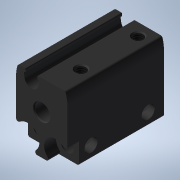
# Autodesk Inventor part: 5267300 AEN-S-6-5-I-A---(highH)
Saved by Autodesk Inventor 2025.1 (Build 291241000, 241)
## iProperties
Category: PARTsolutions
Company: FESTO
Created: 2025-06-16
Part Number: 5267300 AEN-S-6-5-I-A---(highH)
Material: Generic
Catalog Web Link: www.cadenas.de
Description: AEN-S---(H)-Compact cylinder
Vendor: FESTO
Document SubType Name: Modeling
Designer: psAdmin
Manufacturer: FESTO
Mass: 4.06306 g
Surface Area: 29.8936 cm^2
Volume: 4.06306 cm^3
Density: 1 g/cm^3
Appearance: PSOLRGB-175-175-175
PSOL_IDENT_0: {$CADENAS_DATA/23d-libs/festo/parts/a/aen/parts/aen_s_housing.prj},215 {VTYP=3D},{NB=5267300 AEN-S-6
PSOL_IDENT_1: -5-I-A---(highH)},{LINA=5267300 AEN-S-6-5-I-A---(highH)},{NN=AEN-S---(H)},{DATE=04.06.2025 19:32:15}
PSOL_IDENT_2: ,{GEOMDATE=23.08.2023 14:28:27},{VERSION=},{LINEID=30},{WBVAR=LODLEVEL},{WBNUMERIC=}  {NB=5267300 AE
PSOL_IDENT_3: N-S-6-5-I-A---(highH)},{LINA=5267300 AEN-S-6-5-I-A---(highH)},{KT=DUMMY},{TNR=5267300},{TYP=AEN-S-6-
PSOL_IDENT_4: 5-I-A},{LODDEST=mechanical},{LODLEVEL=high},{LODLEVELX='high', 'High', 'medium', 'Medium','low','Low'
PSOL_IDENT_5: },{BAU=S},{KDM=6},{HUB=5},{A=5.000},{SF=3.500},{E1=13.000},{E2=17.500},{ZB=27.500},{ZA=24.500},{L2=8
PSOL_IDENT_6: .100},{L3=10.000},{L4=7.000},{WL=2.700},{T=3.000},{KF=M2.5},{KFD=2.5},{P1=6.000},{P2=4.000},{P3=3.00
PSOL_IDENT_7: 0},{PL1=7.000},{PL2=3.000},{TG=7.000},{D1=5.800},{D2=3.300},{EE=M3},{EED=3.0},{MM=4.000},{WH=3.000}
NB: 5267300 AEN-S-6-5-I-A---(highH)
NN: AEN-S---(H)
NT: Compact cylinder
NBSYN: $TNR. $TYP.---($LODLEVEL.H)
LINA: 5267300 AEN-S-6-5-I-A---(highH)
CATALOG: Festo
TNR: 5267300
TYP: AEN-S-6-5-I-A
LODLEVEL: High
BAU: S
KDM: 6
HUB: 5
A: 5
SF: 3.5
E1: 13
E2: 17.5
ZB: 27.5
ZA: 24.5
L2: 8.1
L3: 10
L4: 7
WL: 2.7
T: 3
KF: M2.5
KFD: 2.5
P1: 6
P2: 4
P3: 3
PL1: 7
PL2: 3
TG: 7
D1: 5.8
D2: 3.3
EE: M3
EED: 3
MM: 4
WH: 3
SUPPLIER: FESTO
ARTICLENO: 5267300 AEN-S-6-5-I-A---(highH)
BOMINFO: 5267300 AEN-S-6-5-I-A---(highH)
CREATOR: CADENAS GmbH
Title: 5267300 AEN-S-6-5-I-A---(highH)
Author: Cadenas PARTsolutions
Comments: Compact cylinder
Autodesk Inventor part; units mm, degrees
sketch "Sketch_1" plane through (0, 0, 0) normal (0, 0, 1) x (1, 0, 0)
  arc A0 (-6.5, -9.5) -> (-6, -10) centre (-6, -9.5) ccw
  line L0 (-6, -10) -> (6, -10)
  arc A1 (6, -10) -> (6.5, -9.5) centre (6, -9.5) ccw
  line L1 (6.5, -9.5) -> (6.5, 4.8)
  arc A2 (6.5, 4.8) -> (6.1481, 7.1467) centre (-1.5, 4.8) ccw
  arc A3 (6.1481, 7.1467) -> (5.6701, 7.5) centre (5.6701, 7) ccw
  line L2 (5.6701, 7.5) -> (-0.9, 7.5)
  arc A4 (-0.9, 7.5) -> (-1.1, 7.3) centre (-0.9, 7.3) ccw
  line L3 (-1.1, 7.3) -> (-1.1, 6.9)
  arc A5 (-1.1, 6.9) -> (-0.8993, 6.7) centre (-0.9, 6.9) ccw
  arc A6 (-0.7, 6.4755) -> (-0.8993, 6.7) centre (-0.8985, 6.5) ccw
  line L4 (-0.7, 6.4755) -> (-0.824, 5.4709)
  arc A7 (-4.376, 5.4709) -> (-0.824, 5.4709) centre (-2.6, 5.69) ccw
  line L5 (-4.376, 5.4709) -> (-4.5, 6.4755)
  arc A8 (-4.3007, 6.7) -> (-4.5, 6.4755) centre (-4.3015, 6.5) ccw
  arc A9 (-4.3007, 6.7) -> (-4.1, 6.9) centre (-4.3, 6.9) ccw
  line L6 (-4.1, 6.9) -> (-4.1, 7.3)
  arc A10 (-4.1, 7.3) -> (-4.3, 7.5) centre (-4.3, 7.3) ccw
  line L7 (-4.3, 7.5) -> (-5.6701, 7.5)
  arc A11 (-5.6701, 7.5) -> (-6.1481, 7.1467) centre (-5.6701, 7) ccw
  arc A12 (-6.1481, 7.1467) -> (-6.5, 4.8) centre (1.5, 4.8) ccw
  line L8 (-6.5, 4.8) -> (-6.5, -9.5)
  constraints: 26 point on circle, 18 end point, 13 centre point
extrude "Extrusion1" add sketch "Sketch_1" against normal blind 24.5
sketch "Sketch_2" plane through (0, 0, 0) normal (0, 0, 1) x (1, 0, 0)
  line L0 (-8.5, -12) -> (8.5, -12)
  line L1 (8.5, -12) -> (8.5, -4.5174)
  line L2 (8.5, -4.5174) -> (6.5, -4.5174)
  arc A0 (5.75, -4.9504) -> (6.5, -4.5174) centre (6, -4.5174) ccw
  line L3 (5.75, -4.9504) -> (4.95, -4.4885)
  arc A1 (4.95, -4.4885) -> (1.2785, -8.8641) centre (3.5, -7) ccw
  line L4 (1.2785, -8.8641) -> (1.5424, -9.1786)
  arc A2 (1.1594, -10) -> (1.5424, -9.1786) centre (1.1594, -9.5) ccw
  line L5 (1.1594, -10) -> (-1.1594, -10)
  arc A3 (-1.5424, -9.1786) -> (-1.1594, -10) centre (-1.1594, -9.5) ccw
  line L6 (-1.5424, -9.1786) -> (-1.2785, -8.8641)
  arc A4 (-1.2785, -8.8641) -> (-4.95, -4.4885) centre (-3.5, -7) ccw
  line L7 (-4.95, -4.4885) -> (-5.75, -4.9504)
  arc A5 (-6.5, -4.5174) -> (-5.75, -4.9504) centre (-6, -4.5174) ccw
  line L8 (-6.5, -4.5174) -> (-8.5, -4.5174)
  line L9 (-8.5, -4.5174) -> (-8.5, -12)
  constraints: 20 end point, 12 point on circle, 6 centre point
extrude "Extrusion2" cut sketch "Sketch_2" against normal blind 3
sketch "Sketch3" plane through (0, 0, -24.5) normal (0, 0, -1) x (-1, 0, 0)
  point P0 (-3.5, -7)
hole "Hole1" at (3.5, -7, -24.5) direction (0, 0, 1) diameter 3.3 depth 24.5
sketch "Sketch4" plane through (0, 0, -24.5) normal (0, 0, -1) x (-1, 0, 0)
  point P0 (3.5, -7)
hole "Hole2" at (-3.5, -7, -24.5) direction (0, 0, 1) diameter 3.3 depth 24.5
sketch "Sketch5" plane through (6.5, -9.5, -24.5) normal (1, 0, 0) x (0, 0, -1)
  point P0 (-18.5, 2.5)
hole "Hole3" at (6.5, -7, -6) direction (-1, 0, 0) diameter 3.3 depth 13
sketch "Sketch6" plane through (6.5, -9.5, -24.5) normal (1, 0, 0) x (0, 0, -1)
  point P0 (-4, 2.5)
hole "Hole4" at (6.5, -7, -20.5) direction (-1, 0, 0) diameter 3.3 depth 13
sketch "Sketch7" plane through (-0.9, 7.5, 0) normal (0, 1, 0) x (1, 0, 0)
  point P0 (3.9, 7)
hole "Hole5" at (3, 7.5, -7) direction (0, -1, 0) diameter 2.459 depth 3.8 countersink diameter 3 countersink angle 90 thread size "M3x0.5" class "6H" standard "ISO Metric profile"
sketch "Sketch8" plane through (-0.9, 7.5, 0) normal (0, 1, 0) x (1, 0, 0)
  point P0 (3.9, 21.5)
hole "Hole6" at (3, 7.5, -21.5) direction (0, -1, 0) diameter 2.459 depth 3.8 countersink diameter 3 countersink angle 90 thread size "M3x0.5" class "6H" standard "ISO Metric profile"
sketch "Sketch_9" plane through (0, 0, 0) normal (1, 0, 0) x (0, 1, 0)
  line L0 (0, -24.5) -> (0, -24.1)
  line L1 (0, -24.1) -> (3.3845, -24.1)
  line L2 (3.3845, -24.1) -> (3.5, -23.9)
  line L3 (3.5, -23.9) -> (3.5, -24.4)
  line L4 (3.5, -24.4) -> (3.6, -24.5)
  line L5 (3.6, -24.5) -> (0, -24.5)
  line L6 (0, -24.5) -> (0, -24.1)
  constraints: 14 end point
revolve "Revolution1" cut sketch "Sketch_9" angle 360 about axis through (0, 0, -24.5) along (0, 0, -1)
sketch "Sketch_10" plane through (0, 0, 0) normal (1, 0, 0) x (0, 1, 0)
  line L0 (0, -22.1) -> (0, 0)
  line L1 (0, 0) -> (2.1732, 0)
  line L2 (2.1732, 0) -> (2, -0.3)
  line L3 (2, -0.3) -> (2, -9)
  line L4 (2, -9) -> (3, -9)
  line L5 (3, -9) -> (3, -22.1)
  line L6 (3, -22.1) -> (0, -22.1)
  line L7 (0, -22.1) -> (0, 0)
  constraints: 16 end point
revolve "Revolution2" cut sketch "Sketch_10" angle 360 about axis through (0, 0, -22.1) along (0, 0, -1)
ref_plane "ANBAU_XY" through (0, 0, 0) normal (0, 0, 1) x (1, 0, 0)
ref_plane "ANBAU_YZ" through (0, 0, 0) normal (1, 0, 0) x (0, 1, 0)
ref_plane "ANBAU_ZX" through (0, 0, 0) normal (0, 1, 0) x (0, 0, 1)
ref_plane "FDT_QSFRONT_XY" through (3, 7.5, -7) normal (0, 1, 0) x (1, 0, 0)
ref_plane "FDT_QSFRONT_YZ" through (3, 7.5, -7) normal (1, 0, 0) x (0, 0, -1)
ref_plane "FDT_QSFRONT_ZX" through (3, 7.5, -7) normal (0, 0, -1) x (0, 1, 0)
ref_plane "FDT_QSREAR_XY" through (3, 7.5, -21.5) normal (0, 1, 0) x (1, 0, 0)
ref_plane "FDT_QSREAR_YZ" through (3, 7.5, -21.5) normal (1, 0, 0) x (0, 0, -1)
ref_plane "FDT_QSREAR_ZX" through (3, 7.5, -21.5) normal (0, 0, -1) x (0, 1, 0)
ref_plane "FDT_SLOT2_XY" through (-2.6, 3.9005, -12.25) normal (0, 1, 0) x (1, 0, 0)
ref_plane "FDT_SLOT2_YZ" through (-2.6, 3.9005, -12.25) normal (1, 0, 0) x (0, 0, -1)
ref_plane "FDT_SLOT2_ZX" through (-2.6, 3.9005, -12.25) normal (0, 0, -1) x (0, 1, 0)
ref_plane "TO_P_XY" through (0, 0, -22.1) normal (0, 0, 1) x (1, 0, 0)
ref_plane "TO_P_YZ" through (0, 0, -22.1) normal (1, 0, 0) x (0, 1, 0)
ref_plane "TO_P_ZX" through (0, 0, -22.1) normal (0, 1, 0) x (0, 0, 1)
body "Solid1"
